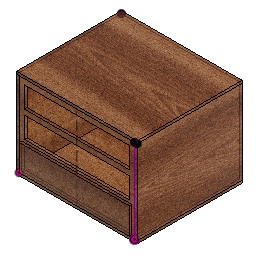
Day21 - Chest of drawers with parameters (Autodesk Fusion 360 design; units mm, degrees)
Autodesk Fusion 360 part; units mm, degrees
sketch "Sketch1" plane through (0, 0, 0) normal (0, 1, 0) x (1, 0, 0)
  line L0 (0, 0) -> (440, 0)
  line L1 (440, 0) -> (440, -320)
  line L2 (440, -320) -> (0, -320)
  line L3 (0, -320) -> (0, 0)
  line L4 (20, -100) -> (420, -100)
  line L5 (420, -100) -> (420, -20)
  line L6 (420, -20) -> (20, -20)
  line L7 (20, -20) -> (20, -100)
  line L8 (220, 0) -> (220, -320) construction
  line L9 (430, -10) -> (10, -10)
  line L10 (10, -10) -> (10, -110)
  line L11 (10, -110) -> (430, -110)
  line L12 (430, -110) -> (430, -10)
  dimension "d6" = 440
  dimension "d7" = 320
  dimension "d8" = 80
  dimension "d9" = 400
  dimension "d10" = 20
  dimension "d33" = 10
  measures "d6" distance of L0.start
  measures "d9" distance of L0.start
  measures "d10" distance of L0 L6
  measures "d33" distance of L6
extrude "Extrude1" add sketch "Sketch1" along normal blind 10 contours L0 L1 L2 L3 | L4 L5 L6 L7 | L9 L10 L11 L12 makes body 1
extrude "Extrude2" cut sketch "Sketch1" along normal up to surface (10 mm away) contours L4 L5 L6 L7 bodies 1
pattern_linear "R-Pattern1" count 3 spacing 100 along (0, 0, 1) of "Extrude2"
sketch "Sketch2" plane through (440, 0, 0) normal (1, 0, 0) x (0, 1, 0)
  line L0 (0, 0) -> (0, 320)
  line L1 (0, 320) -> (400, 320)
  line L2 (400, 320) -> (400, 0)
  line L3 (400, 0) -> (0, 0)
  line L4 (0, 0) -> (0, 320)
  dimension "d19" = 400
extrude "Extrude3" add sketch "Sketch2" along normal blind 10 separate body makes body 2
extrude "Extrude4" add sketch "Sketch2" against normal blind 10 from surface at -440 separate body makes body 3
extrude "Extrude5" add sketch "Sketch1" against normal blind 10 from surface at 400 separate body contours L0 L1 L2 L3 | L4 L5 L6 L7 | L9 L10 L11 L12 makes body 4
sketch "Sketch3" plane through (0, 0, 320) normal (0, 0, 1) x (-1, 0, 0)
  line L0 (10, -400) -> (-450, -400)
  line L1 (-450, -400) -> (-450, 0)
  line L2 (-450, 0) -> (10, 0)
  line L3 (10, 0) -> (10, -400)
extrude "Extrude6" add sketch "Sketch3" along normal blind 10 separate body makes body 5
extrude "Extrude7" add sketch "Sketch3" against normal blind 10 from surface at -320 separate body makes body 6
extrude "Extrude8" add sketch "Sketch1" against normal blind 10 separate body contours L4 L5 L6 L7 | L9 L10 L11 L12 makes body 7
equation "numdrawers = 3"
equation "thickness = 10 mm"
equation "space = thickness * 2"
equation "drheight = 80 mm"
equation "drlong = 400 mm"
equation "d6 = drlong + space * 2"
equation "d7 = numdrawers * ( drheight + space ) + space"
equation "d8 = drheight"
equation "d9 = drlong"
equation "d10 = space"
equation "d11 = thickness"
equation "d15 = numdrawers"
equation "d17 = space + drheight"
equation "d19 = drlong"
equation "d20 = thickness"
equation "d23 = -thickness"
equation "d26 = -thickness"
equation "d28 = thickness"
equation "d31 = -thickness"
equation "d33 = thickness"
equation "d34 = -thickness"
